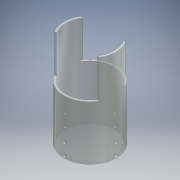
# Autodesk Inventor part: outsideCover
Saved by Autodesk Inventor 2016 (Build 200138000, 138)
## iProperties
Created: 2016-10-27
Part Number: outsideCover
Material: ガラス
Document SubType Name: Modeling
Designer: Daisuke
Density: 2.18 g/cm^3
Appearance: クリア
Author: Daisuke
Autodesk Inventor part; units mm, degrees
ref_plane "XY Plane" through (0, 0, 0) normal (0, 0, 1) x (1, 0, 0)
sketch "スケッチ1" plane through (0, 0, 0) normal (0, 0, 1) x (1, 0, 0)
  circle A0 centre (0, 0) radius 51
  circle A1 centre (0, 0) radius 55
  line L0 (0, 0) -> (47.6314, 27.5) construction
  line L1 (0, 0) -> (55, 0) construction
  line L2 (0, 0) -> (-47.6314, 27.5) construction
  line L3 (0, 0) -> (55, 0) construction
  dimension "d0" = 102
  dimension "d1" = 110
  dimension "d2" = 30
  dimension "d3" = 150
  constraints: 8 end point, 2 centre point, 2 coincident, 2 equal length, 2 horizontal, 2 point on circle
  measures "d0" diameter of A0
  measures "d1" diameter of A1
  measures "d2" angle of L1 L0
  measures "d3" angle of L3 L2
extrude "押し出し1" add sketch "スケッチ1" along normal blind 20
sketch "スケッチ2" plane through (0, 0, 20) normal (0, 0, 1) x (1, 0, 0)
  line L0 (0, 0) -> (47.6314, 27.5) construction
  circle A0 centre (0, 0) radius 55 construction
  line L1 (0, 0) -> (55, 0) construction
  line L2 (0, 0) -> (-47.6314, 27.5) construction
  line L3 (0, 0) -> (55, 0) construction
  line L4 (0, 0) -> (47.6314, -27.5) construction
  line L5 (0, 0) -> (55, 0) construction
  line L6 (0, 0) -> (-47.6314, -27.5) construction
  line L7 (0, 0) -> (55, 0) construction
  arc A1 (-47.6314, 27.5) -> (-47.6314, -27.5) centre (0, 0) ccw
  arc A2 (47.6314, -27.5) -> (47.6314, 27.5) centre (0, 0) ccw
  arc A3 (-42.9506, 27.5) -> (-42.9506, -27.5) centre (0, 0) ccw
  arc A4 (42.9506, -27.5) -> (42.9506, 27.5) centre (0, 0) ccw
  line L8 (-47.6314, 27.5) -> (-42.9506, 27.5)
  line L9 (42.9506, 27.5) -> (47.6314, 27.5)
  line L10 (-47.6314, -27.5) -> (-42.9506, -27.5)
  line L11 (42.9506, -27.5) -> (47.6314, -27.5)
  dimension "d6" = 30
  dimension "d7" = 150
  dimension "d43" = 30
  dimension "d44" = 150
  dimension "d55" = 51
  dimension "d56" = 51
  constraints: 24 end point, 12 point on circle, 4 centre point, 4 equal length, 4 horizontal, 2 coincident
  measures "d6" angle of L1 L0
  measures "d7" angle of L3 L2
  measures "d43" angle of L4 L5
  measures "d44" angle of L6 L7
  measures "d55" radius of A3
  measures "d56" radius of A4
ref_plane "作業平面1" through (55, 0, 0) normal (1, 0, 0) x (0, 1, 0)
ref_plane "作業平面2" through (-55, 0, 0) normal (1, 0, 0) x (0, 1, 0)
ref_plane "作業平面3" through (0, 55, 0) normal (0, 1, 0) x (-1, 0, 0)
ref_plane "作業平面4" through (0, -55, 0) normal (0, 1, 0) x (-1, 0, 0)
sketch "スケッチ3" plane through (55, 0, 0) normal (1, 0, 0) x (0, 1, 0)
  line L0 (0, 0) -> (0, 4) construction
  circle A0 centre (0, 4) radius 1.5
  dimension "d14" = 4
  dimension "d15" = 3
  constraints: 2 end point, 1 centre point, 1 coincident, 1 vertical
  measures "d14" distance of L0.start L0.end
  measures "d15" diameter of A0
extrude "押し出し3" cut sketch "スケッチ3" against normal blind 6
sketch "スケッチ4" plane through (0, 55, 0) normal (0, 1, 0) x (-1, 0, 0)
  line L0 (0, 0) -> (0, 4) construction
  circle A0 centre (0, 4) radius 1.5
  dimension "d18" = 4
  dimension "d19" = 3
  constraints: 2 end point, 1 centre point, 1 coincident, 1 vertical
  measures "d18" distance of L0.start L0.end
  measures "d19" diameter of A0
extrude "押し出し4" cut sketch "スケッチ4" against normal blind 6
sketch "スケッチ5" plane through (-55, 0, 0) normal (1, 0, 0) x (0, 1, 0)
  line L0 (0, 0) -> (0, 4) construction
  circle A0 centre (0, 4) radius 1.5
  dimension "d22" = 4
  dimension "d23" = 3
  constraints: 2 end point, 1 centre point, 1 coincident, 1 vertical
  measures "d22" distance of L0.start L0.end
  measures "d23" diameter of A0
extrude "押し出し5" cut sketch "スケッチ5" along normal blind 6
sketch "スケッチ6" plane through (0, -55, 0) normal (0, 1, 0) x (-1, 0, 0)
  line L0 (0, 0) -> (0, 4) construction
  circle A0 centre (0, 4) radius 1.5
  dimension "d26" = 4
  dimension "d27" = 3
  constraints: 2 end point, 1 centre point, 1 coincident, 1 vertical
  measures "d26" distance of L0.start L0.end
  measures "d27" diameter of A0
extrude "押し出し6" cut sketch "スケッチ6" along normal blind 6
ref_plane "作業平面5" through (55, 0, 0) normal (1, 0, 0) x (0, 1, 0)
extrude "押し出し9" add sketch "スケッチ2" along normal blind 150
sketch "スケッチ9" plane through (55, 0, 0) normal (1, 0, 0) x (0, 1, 0)
  line L0 (0, 0) -> (0, 12) construction
  line L1 (0, 12) -> (-3.5, 12) construction
  line L2 (-3.5, 12) -> (-13.5, 12)
  line L3 (-13.5, 12) -> (-13.5, 20)
  line L4 (-13.5, 20) -> (-3.5, 20)
  line L5 (-3.5, 20) -> (-3.5, 12)
  dimension "d49" = 12
  dimension "d50" = 3.5
  dimension "d51" = 10
  dimension "d52" = 8
  constraints: 12 end point, 2 horizontal, 2 parallel, 1 perpendicular, 1 vertical
  measures "d49" distance of L0.start L0.end
  measures "d50" distance of L0.end L1.end
  measures "d51" distance of L3.end L4.end
  measures "d52" distance of L2.end L3.end
sketch "スケッチ10" plane through (0, 0, 0) normal (0, 0, -1) x (-1, 0, 0)
  circle A0 centre (0, 0) radius 51
  circle A1 centre (0, 0) radius 55
  constraints: 2 centre point, 2 coincident
extrude "押し出し12" add sketch "スケッチ10" along normal blind 25
sketch "スケッチ11" plane through (0, 0, 20) normal (0, 0, 1) x (1, 0, 0)
  line L0 (47.6314, -27.5) -> (42.9506, -27.5) construction
  line L1 (0, 0) -> (47.6314, -27.5) construction
  line L2 (0, 0) -> (55, 0) construction
  line L3 (0, 0) -> (-47.6314, -27.5) construction
  line L4 (0, 0) -> (55, 0) construction
  arc A0 (-47.6314, -27.5) -> (47.6314, -27.5) centre (0, 0) ccw
  arc A1 (-42.9506, -27.5) -> (42.9506, -27.5) centre (0, 0) ccw projected
  arc A2 (42.9506, -27.5) -> (42.9506, -27.5) centre (0, 0) ccw
  line L5 (-47.6314, -27.5) -> (-42.9506, -27.5)
  line L6 (42.9506, -27.5) -> (47.6314, -27.5)
  dimension "d59" = 30
  dimension "d60" = 150
  constraints: 12 end point, 6 point on circle, 2 centre point, 2 coincident, 2 equal length, 2 horizontal
  measures "d59" angle of L1 L2
  measures "d60" angle of L3 L4
extrude "押し出し13" add sketch "スケッチ11" along normal blind 70 contours L5 A1 L6 A0
sketch "スケッチ12" plane through (55, 0, 0) normal (1, 0, 0) x (0, 1, 0)
  line L0 (0, 0) -> (0, -21) construction
  line L1 (51, -25) -> (-51, -25) construction
  circle A0 centre (0, -21) radius 1.5
  dimension "d63" = 21
  dimension "d64" = 3
  constraints: 2 end point, 1 centre point, 1 coincident, 1 perpendicular
  measures "d63" distance of L0.start L0.end
  measures "d64" diameter of A0
extrude "押し出し14" cut sketch "スケッチ12" against normal blind 5
sketch "スケッチ13" plane through (-55, 0, 0) normal (1, 0, 0) x (0, 1, 0)
  line L0 (0, 0) -> (0, -21) construction
  circle A0 centre (0, -21) radius 1.5
  dimension "d67" = 21
  dimension "d68" = 3
  constraints: 2 end point, 1 centre point, 1 coincident, 1 vertical
  measures "d67" distance of L0.start L0.end
  measures "d68" diameter of A0
extrude "押し出し15" cut sketch "スケッチ13" along normal blind 5
sketch "スケッチ14" plane through (0, 55, 0) normal (0, 1, 0) x (-1, 0, 0)
  line L0 (0, 0) -> (0, -21) construction
  circle A0 centre (0, -21) radius 1.5
  dimension "d71" = 21
  dimension "d72" = 3
  constraints: 2 end point, 1 centre point, 1 coincident, 1 vertical
  measures "d71" distance of L0.start L0.end
  measures "d72" diameter of A0
extrude "押し出し16" cut sketch "スケッチ14" against normal blind 5
sketch "スケッチ15" plane through (0, -55, 0) normal (0, 1, 0) x (-1, 0, 0)
  line L0 (0, 0) -> (0, -21) construction
  circle A0 centre (0, -21) radius 1.5
  dimension "d75" = 21
  dimension "d76" = 3
  constraints: 2 end point, 1 centre point, 1 coincident, 1 vertical
  measures "d75" distance of L0.start L0.end
  measures "d76" diameter of A0
extrude "押し出し17" cut sketch "スケッチ15" along normal blind 5
sketch "スケッチ16" plane through (0, 0, 20) normal (0, 0, 1) x (1, 0, 0)
  line L0 (-47.6314, 27.5) -> (-42.9506, 27.5) construction
  line L1 (0, 0) -> (-47.6314, 27.5) construction
  line L2 (0, 0) -> (-55, 0) construction
  line L3 (0, 0) -> (47.6314, 27.5) construction
  line L4 (0, 0) -> (-55, 0) construction
  arc A0 (47.6314, 27.5) -> (-47.6314, 27.5) centre (0, 0) ccw
  arc A1 (42.9506, 27.5) -> (-42.9506, 27.5) centre (0, 0) ccw
  arc A2 (-42.9506, 27.5) -> (-42.9506, 27.5) centre (0, 0) ccw
  line L5 (47.6314, 27.5) -> (42.9506, 27.5)
  line L6 (-42.9506, 27.5) -> (-47.6314, 27.5)
  dimension "d79" = 30
  dimension "d80" = 150
  constraints: 14 end point, 8 point on circle, 3 centre point, 2 coincident, 2 equal length
  measures "d79" angle of L1 L2
  measures "d80" angle of L3 L4
extrude "押し出し18" add sketch "スケッチ16" along normal blind 70 contours L5 A1 L6 A0
sketch "スケッチ17" plane through (55, 0, 0) normal (1, 0, 0) x (0, 1, 0)
  line L0 (0, 0) -> (0, 4) construction
  line L1 (0, 0) -> (0, -21) construction
  circle A0 centre (0, -21) radius 2.5
  circle A1 centre (0, 4) radius 2.5
  dimension "d83" = 4
  dimension "d84" = 21
  dimension "d85" = 5
  dimension "d86" = 5
  constraints: 4 end point, 2 centre point, 2 coincident, 2 vertical
  measures "d83" distance of L0.start L0.end
  measures "d84" distance of L0.start L1.end
  measures "d85" diameter of A0
  measures "d86" diameter of A1
extrude "押し出し19" cut sketch "スケッチ17" against normal blind 3
sketch "スケッチ18" plane through (-55, 0, 0) normal (1, 0, 0) x (0, 1, 0)
  line L0 (0, 0) -> (0, 4) construction
  line L1 (0, 0) -> (0, -21) construction
  circle A0 centre (0, -21) radius 2.5
  circle A1 centre (0, 4) radius 2.5
  dimension "d89" = 4
  dimension "d90" = 21
  dimension "d91" = 5
  dimension "d92" = 5
  constraints: 4 end point, 2 centre point, 2 coincident, 2 vertical
  measures "d89" distance of L0.start L0.end
  measures "d90" distance of L0.start L1.end
  measures "d91" diameter of A0
  measures "d92" diameter of A1
extrude "押し出し20" cut sketch "スケッチ18" along normal blind 3
sketch "スケッチ19" plane through (0, 55, 0) normal (0, 1, 0) x (-1, 0, 0)
  line L0 (0, 0) -> (0, 4) construction
  line L1 (0, 0) -> (0, -21) construction
  circle A0 centre (0, 4) radius 2.5
  circle A1 centre (0, -21) radius 2.5
  dimension "d95" = 4
  dimension "d96" = 21
  dimension "d97" = 5
  dimension "d98" = 5
  constraints: 4 end point, 2 centre point, 2 coincident, 2 vertical
  measures "d95" distance of L0.start L0.end
  measures "d96" distance of L0.start L1.end
  measures "d97" diameter of A0
  measures "d98" diameter of A1
extrude "押し出し21" cut sketch "スケッチ19" against normal blind 3
sketch "スケッチ20" plane through (0, -55, 0) normal (0, 1, 0) x (-1, 0, 0)
  line L0 (0, 0) -> (0, 4) construction
  circle A0 centre (0, -21) radius 1.5 construction
  line L1 (0, 0) -> (0, -21) construction
  circle A1 centre (0, -21) radius 2.5
  circle A2 centre (0, 4) radius 2.5
  dimension "d101" = 4
  dimension "d102" = 21
  dimension "d103" = 5
  dimension "d104" = 5
  constraints: 4 end point, 2 centre point, 2 coincident, 2 vertical
  measures "d101" distance of L0.start L0.end
  measures "d102" distance of L0.start L1.end
  measures "d103" diameter of A1
  measures "d104" diameter of A2
extrude "押し出し22" cut sketch "スケッチ20" along normal blind 3
